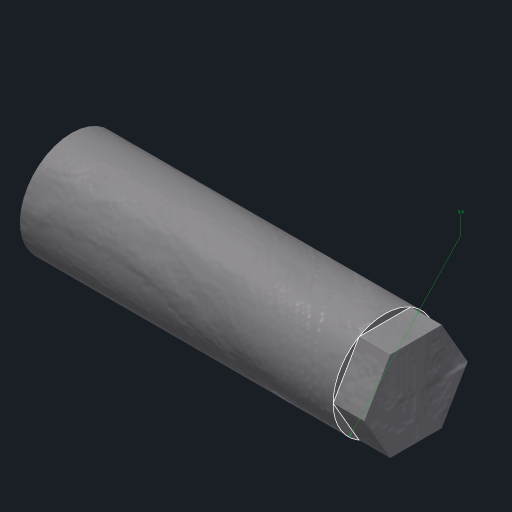
# Autodesk Inventor part: EJE
Saved by Autodesk Inventor 2024.3 (Build 283343000, 343)
## iProperties
Created: 2024-06-30
Part Number: EJE
Material: Steel, Mild, Welded
Document SubType Name: Modeling
Designer: Niler
Density: 7.85 g/cm^3
Appearance: Weld - Steel Mild
Author: Niler
Autodesk Inventor part; units mm, degrees
ref_plane "YZ Plane" through (0, 0, 0) normal (1, 0, 0) x (0, 1, 0)
ref_plane "XZ Plane" through (0, 0, 0) normal (0, 1, 0) x (-1, 0, 0)
ref_plane "XY Plane" through (0, 0, 0) normal (0, 0, 1) x (1, 0, 0)
sketch "Sketch1" plane through (0, 0, 0) normal (1, 0, 0) x (0, 1, 0)
  line L0 (0, -4.95) -> (-4.2868, -2.475)
  line L1 (-4.2868, -2.475) -> (-4.2868, 2.475)
  line L2 (-4.2868, 2.475) -> (0, 4.95)
  line L3 (0, 4.95) -> (4.2868, 2.475)
  line L4 (4.2868, 2.475) -> (4.2868, -2.475)
  line L5 (4.2868, -2.475) -> (0, -4.95)
  circle A0 centre (0, 0) radius 4.95
  dimension "d0" = 9.9
  constraints: 12 end point, 2 coincident, 1 vertical alignment, 16 other
extrude "Extrusion1" add sketch "Sketch1" along normal blind 3 contours L0 L1 L2 L3 L4 L5
extrude "Extrusion2" add sketch "Sketch1" against normal blind 30
body "Solid1"
